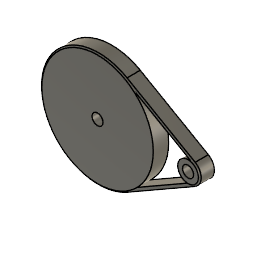
Parametric_ClosedLoop_BeltGenerator_NoTeeth (Autodesk Fusion 360 design; units mm, degrees)
Autodesk Fusion 360 part; units mm, degrees
note: some values were not read from the file. Set by a fixed rule: which sketch regions a step uses.
sketch "Sketch1" plane through (0, 0, 0) normal (0, 1, 0) x (1, 0, 0) in component "Pulley1"
  line L0 (-20.479, 0) -> (20.479, 0)
  circle A0 centre (-20.479, 0) radius 25.2108
  circle A1 centre (-20.479, 0) radius 24.4608
  line L1 (-20.479, 0) -> (-20.479, -25.2108) construction
  line L2 (-20.479, 0) -> (-18.501, -25.1331) construction
  circle A2 centre (-20.479, 0) radius 25.0608 construction
  circle A3 centre (-20.479, 0) radius 2.5
  dimension "d133" = 40.958
  dimension "d134" = 50.4216
  dimension "d135" = -0.75
  dimension "d136" = 4.5
  dimension "d142" = 5
  constraint horizontal L0
  constraint midpoint origin L0
  constraint coincident L0.start A0.centre
  constraint coincident A0 L1.end
  constraint perpendicular L0 L1
  constraint coincident A0 L2.end
  constraint concentric A0 A3
  measures "d133" distance of L0.start L0.end
  measures "d134" diameter of A0
  measures "d136" angle of L1 L2
  measures "d142" diameter of A3
extrude "Extrude2" add sketch "Sketch1" along normal mid plane 7 contours A0 | A1 makes body 1 in component "Pulley1"
sketch "Sketch1 (2)" plane through (0, 0, 0) normal (0, 1, 0) x (1, 0, 0) in component "Pulley2"
  line L0 (20.479, 0) -> (-20.479, 0)
  circle A0 centre (20.479, 0) radius 4.839 construction
  circle A1 centre (20.479, 0) radius 4.089
  circle A2 centre (20.479, 0) radius 4.689
  line L1 (20.479, 0) -> (20.479, -4.839) construction
  line L2 (20.479, 0) -> (18.6272, -4.4706) construction
  line L3 (20.479, -4.089) -> (20.479, -4.644) construction
  line L4 (18.9142, -3.7777) -> (18.7018, -4.2905) construction
  circle A3 centre (20.479, 0) radius 2.5
  dimension "d149" = 40.958
  dimension "d150" = 9.6779
  dimension "d151" = -0.75
  dimension "d153" = 22.5
  dimension "d187" = 0.555
  dimension "d188" = 0.555
  dimension "d196" = 5
  constraint horizontal L0
  constraint midpoint origin L0
  constraint coincident L0.start A0.centre
  constraint coincident A0 L1.end
  constraint vertical L1
  constraint coincident A0 L2.end
  constraint coincident A1 L3.start
  constraint coincident L1 L3.start
  constraint parallel L1 L3
  constraint coincident L2 L4.start
  constraint coincident A1 L4.start
  constraint parallel L2 L4
  constraint concentric A0 A3
  measures "d149" distance of L0.start L0.end
  measures "d150" diameter of A0
  measures "d153" angle of L1 L2
  measures "d187" distance of L3.start L3.end
  measures "d188" distance of L4.start L4.end
  measures "d196" diameter of A3
sketch "Sketch2" plane through (0, 0, 0) normal (0, 1, 0) x (1, 0, 0) in component "Belt"
  line L0 (20.479, 0) -> (-20.479, 0)
  circle A0 centre (-20.479, 0) radius 25.2108 construction
  line L1 (-20.479, 0) -> (-20.479, -25.2108) construction
  circle A1 centre (-20.479, 0) radius 24.4608 construction
  circle A2 centre (20.479, 0) radius 5.093 construction
  line L2 (62.777, 18.3802) -> (-7.8132, -22.0915) construction
  line L3 (39.5189, -5.0456) -> (-31.5457, 35.6981) construction
  line L4 (23.0121, -4.4183) -> (-7.8132, -22.0915)
  line L5 (-7.8132, 22.0915) -> (23.0121, 4.4183)
  arc A3 (23.0121, -4.4183) -> (23.0121, 4.4183) centre (20.479, 0) ccw
  arc A4 (-7.8132, 22.0915) -> (-7.8132, -22.0915) centre (-20.479, 0) ccw
  arc A5 (-7.6262, 22.4177) -> (-7.6261, -22.4177) centre (-20.479, 0) ccw
  line L6 (23.1991, -4.7445) -> (-7.6261, -22.4177)
  arc A6 (23.1991, -4.7445) -> (23.1992, 4.7445) centre (20.479, 0) ccw
  line L7 (-7.6262, 22.4177) -> (23.1992, 4.7445)
  line L8 (22.5128, -3.5473) -> (-8.3125, -21.2205)
  arc A7 (-8.3126, 21.2205) -> (-8.3125, -21.2205) centre (-20.479, 0) ccw
  line L9 (-8.3126, 21.2205) -> (22.5128, 3.5473)
  arc A8 (22.5128, -3.5473) -> (22.5128, 3.5473) centre (20.479, 0) ccw
  line L10 (22.8361, -4.1112) -> (-7.9892, -21.7844)
  arc A9 (-7.9893, 21.7844) -> (-7.9892, -21.7844) centre (-20.479, 0) ccw
  line L11 (-7.9893, 21.7844) -> (22.8361, 4.1112)
  arc A10 (22.8361, -4.1112) -> (22.8361, 4.1112) centre (20.479, 0) ccw
  point P0 (-23.0331, -25.0158)
  dimension "d165" = 40.958
  dimension "d166" = 50.4216
  dimension "d167" = -0.75
  dimension "d171" = 50.9296
  dimension "d172" = 10.1859
  dimension "d174" = 81.916
  dimension "d177" = -0.354
  constraint horizontal L0
  constraint midpoint origin L0
  constraint coincident L0.end A0.centre
  constraint coincident A0 L1.end
  constraint vertical L1
  constraint concentric A0 A4
  constraint coincident L0.start A2.centre
  constraint tangent L2 A4
  constraint tangent A2 L2
  constraint tangent L3 A4
  constraint tangent A2 L3
  constraint coincident A2 L4.start
  constraint coincident L2 L4.start
  constraint coincident L3 L5.start
  constraint coincident A2 L5.end
  constraint tangent A2 L5
  constraint tangent L3 A3
  measures "d165" distance of L0.start L0.end
  measures "d166" diameter of A0
  measures "d171" diameter of A4
  measures "d172" diameter of A2
  measures "d174" distance of L3.start L3.end
extrude "Extrude2'" add sketch "Sketch2" along normal mid plane 6 separate body contours L4 L5 A3 A4 | A5 L6 A6 L7 | L10 A9 L11 A10 makes body 2 in component "Belt"
extrude "Extrude4" add sketch "Sketch1 (2)" along normal mid plane 7 separate body contours A1 | A2 makes body 3 in component "Pulley2"
component "Pulley1" placed x (1, 0, 0) y (0, 1, 0) z (0, 0, 1) at (0, 0, 0)
component "Pulley2" placed x (1, 0, 0) y (0, 1, 0) z (0, 0, 1) at (0, 0, 0)
component "Belt" placed x (1, 0, 0) y (0, 1, 0) z (0, 0, 1) at (0, 0, 0)
equation "Pulley1ToothCount = 80"
equation "Pulley2ToothCount = 16"
equation "R1 = ( D1 / 2 )"
equation "R2 = ( D2 / 2 )"
equation "varA = ( L - ( 1.57 * ( D1 + D2 ) ) )"
equation "D1 = ( ( 2 * Pulley1ToothCount ) / 3.14159 )"
equation "D2 = ( ( 2 * Pulley2ToothCount ) / 3.14159 )"
equation "L = 188"
equation "varB = pow(( D2 - D1 ); 2)"
equation "C2C = ( ( varA + sqrt(pow(varA; 2) - 2 * varB) ) / 4 ) * 1 mm"
equation "beltThickness = 1.38 mm"
equation "rearBeltThickness = beltThickness - 1.004 mm"
equation "frontBeltThickness = beltThickness - 0.376 mm"
equation "beltWidth = 6 mm"
equation "U = 0.254 mm"
equation "ToothHeight = -0.75 mm"
equation "OD1 = ( D1 * mm ) - ( 2 * U )"
equation "OD2 = ( D2 * mm ) - ( 2 * U )"
equation "toothD = ( 0.555 * 2 ) * 1 mm"
equation "pulleyToothRound = ( 0.15 * 2 ) * 1 mm"
equation "pulleyWidth = beltWidth + 1 mm"
equation "boreID = 5 mm"
equation "toothPD = 0.15 mm"
equation "RD1 = ( ( 360 / Pulley1ToothCount ) * 1 deg )"
equation "RD2 = ( ( 360 / Pulley2ToothCount ) * 1 deg )"
equation "d133 = C2C"
equation "d134 = OD1"
equation "d135 = ToothHeight"
equation "d136 = RD1"
equation "d137 = -toothPD"
equation "d147 = pulleyWidth"
equation "d149 = C2C"
equation "d150 = OD2"
equation "d151 = ToothHeight"
equation "d152 = -toothPD"
equation "d153 = RD2"
equation "d165 = C2C"
equation "d166 = OD1"
equation "d167 = ToothHeight"
equation "d171 = D1 * mm"
equation "d172 = D2 * mm"
equation "d174 = C2C * 2"
equation "d175 = -rearBeltThickness"
equation "d176 = -frontBeltThickness"
equation "d177 = -frontBeltThickness + 0.65 mm"
equation "d182 = beltWidth"
equation "d187 = toothD / 2"
equation "d188 = toothD / 2"
equation "d197 = pulleyWidth"
